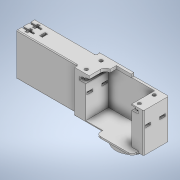
# Autodesk Inventor part: мотор_плеча_2.1-локтя_1
Saved by Autodesk Inventor 2022 (Build 260153000, 153)
## iProperties
Created: 2022-12-03
Part Number: мотор_плеча_2.1-локтя_1
Material: Типовые
Document SubType Name: Modeling
Designer: Папа
Density: 1 g/cm^3
Appearance: По умолчанию
Author: Папа
Autodesk Inventor part; units mm, degrees
ref_plane "YZ Plane" through (0, 0, 0) normal (1, 0, 0) x (0, 1, 0)
ref_plane "XZ Plane" through (0, 0, 0) normal (0, 1, 0) x (-1, 0, 0)
ref_plane "XY Plane" through (0, 0, 0) normal (0, 0, 1) x (1, 0, 0)
sketch "Эскиз1" plane through (0, 0, 0) normal (0, 1, 0) x (-1, 0, 0)
  line L0 (0, 0) -> (-59.05, 0)
  line L1 (-59.05, 0) -> (-59.05, -29.25)
  line L2 (-59.05, -29.25) -> (0, -29.25)
  line L3 (0, -29.25) -> (0, 0)
  line L4 (-74.05, 3) -> (15, 3)
  line L5 (15, 3) -> (15, -32.25)
  line L6 (15, -32.25) -> (-74.05, -32.25)
  line L7 (-74.05, -32.25) -> (-74.05, 3)
  line L8 (-74.05, 3) -> (15, -32.25) construction
  line L9 (15, 3) -> (-74.05, -32.25) construction
  line L10 (0, -29.25) -> (-59.05, 0) construction
  line L11 (0, 0) -> (-59.05, -29.25) construction
  line L12 (15, 0) -> (-74.05, 0)
  point P0 (-29.525, -14.625)
  point P1 (-29.525, -14.625)
  point P2 (-59.05, 0)
  point P3 (-59.05, 0)
  point P4 (0, 0)
  dimension "d0" = 29.25
  dimension "d1" = 59.05
  dimension "d2" = 15
  dimension "d3" = 3
  constraints: 26 end point, 4 midpoint, 4 parallel, 3 point on line, 2 horizontal, 2 perpendicular, 1 collinear
  measures "d0" distance of L2.end L0.start
  measures "d1" distance of L1.end L2.end
  measures "d2" distance between parallel lines of L3 L5
  measures "d3" distance between parallel lines of L6 L2
extrude "Выдавливание1" add sketch "Эскиз1" along normal blind 41 contours L12 L5 L6 L7 L1 L2 L3
sketch "Эскиз2" plane through (0, 0, 0) normal (0, -1, 0) x (1, 0, 0)
  line L0 (74.05, 0) -> (74.05, -32.25) projected
  line L1 (-15, -32.25) -> (-15, 0) projected
  line L2 (74.05, 0) -> (-15, 0)
  line L3 (-15, 0) -> (-15, -32.25)
  line L4 (-15, -32.25) -> (74.05, -32.25)
  line L5 (74.05, -32.25) -> (74.05, 0)
  point P0 (0, 0)
  constraints: 8 end point, 2 parallel, 1 horizontal, 1 perpendicular
extrude "Выдавливание2" add sketch "Эскиз2" along normal blind 2
sketch "Эскиз3" plane through (0, 41, 0) normal (0, 1, 0) x (1, 0, 0)
  circle A0 centre (-4.475, 5.225) radius 2.1
  circle A1 centre (-4.475, 24.225) radius 2.1
  circle A2 centre (63.525, 24.225) radius 2.1
  circle A3 centre (63.525, 5.225) radius 2.1
  line L0 (59.05, 29.25) -> (59.05, 0) construction
  line L1 (0, 0) -> (0, 29.25) construction
  line L2 (59.05, 29.25) -> (0, 29.25) construction
  line L3 (0, 29.25) -> (0, 0.2) construction
  line L4 (0, 0.2) -> (59.05, 0.2) construction
  line L5 (59.05, 0.2) -> (59.05, 29.25) construction
  line L6 (0, 0) -> (59.05, 0) construction
  line L7 (59.05, 0) -> (59.05, 0.2) construction
  line L8 (59.05, 0.2) -> (0, 0.2) construction
  line L9 (0, 0.2) -> (0, 0) construction
  line L10 (0, 0.2) -> (59.05, 29.25) construction
  line L11 (59.05, 0.2) -> (0, 29.25) construction
  line L12 (-4.475, 5.225) -> (63.525, 5.225) construction
  line L13 (63.525, 5.225) -> (63.525, 24.225) construction
  line L14 (63.525, 24.225) -> (-4.475, 24.225) construction
  line L15 (-4.475, 24.225) -> (-4.475, 5.225) construction
  line L16 (-4.475, 5.225) -> (63.525, 24.225) construction
  line L17 (-4.475, 24.225) -> (63.525, 5.225) construction
  point P0 (29.525, 14.725)
  dimension "d8" = 4.2
  dimension "d70" = 0.2
  dimension "d72" = 19
  dimension "d73" = 68
  constraints: 32 end point, 6 parallel, 4 centre point, 3 equal radius, 3 horizontal, 3 perpendicular, 2 coincident, 2 midpoint, 1 point on line
  measures "d8" diameter of A0
  measures "d70" distance between parallel lines of L4 L6
  measures "d72" distance of L13.end A3.centre
  measures "d73" distance of L13.end L14.end
extrude "Выдавливание3" cut sketch "Эскиз3" against normal blind 20
ref_plane "РабПлоскость1" through (0, 31, 0) normal (0, 1, 0) x (1, 0, 0)
sketch "Эскиз4" plane through (0, 31, 0) normal (0, 1, 0) x (1, 0, 0)
  circle A0 centre (63.525, 24.225) radius 2.1 projected
  line L0 (65.589, 27.8) -> (67.6531, 24.225)
  line L1 (67.6531, 24.225) -> (65.589, 20.65)
  line L2 (65.589, 20.65) -> (61.461, 20.65)
  line L3 (61.461, 20.65) -> (59.3969, 24.225)
  line L4 (59.3969, 24.225) -> (61.461, 27.8)
  line L5 (61.461, 27.8) -> (65.589, 27.8)
  circle A1 centre (-4.475, 24.225) radius 2.1 construction
  circle A2 centre (63.525, 5.225) radius 2.1 projected
  line L6 (-4.475, 24.225) -> (63.525, 24.225) construction
  line L7 (63.525, 24.225) -> (63.525, 5.225) construction
  line L8 (63.525, 5.225) -> (-4.475, 5.225) construction
  line L9 (-4.475, 5.225) -> (-4.475, 24.225) construction
  line L10 (-2.411, 27.8) -> (-0.3469, 24.225)
  line L11 (-0.3469, 24.225) -> (-2.411, 20.65)
  line L12 (-2.411, 20.65) -> (-6.539, 20.65)
  line L13 (-6.539, 20.65) -> (-8.6031, 24.225)
  line L14 (-8.6031, 24.225) -> (-6.539, 27.8)
  line L15 (-6.539, 27.8) -> (-2.411, 27.8)
  line L16 (65.589, 8.8) -> (67.6531, 5.225)
  line L17 (67.6531, 5.225) -> (65.589, 1.65)
  line L18 (65.589, 1.65) -> (61.461, 1.65)
  line L19 (61.461, 1.65) -> (59.3969, 5.225)
  line L20 (59.3969, 5.225) -> (61.461, 8.8)
  line L21 (61.461, 8.8) -> (65.589, 8.8)
  line L22 (-2.411, 8.8) -> (-0.3469, 5.225)
  line L23 (-0.3469, 5.225) -> (-2.411, 1.65)
  line L24 (-2.411, 1.65) -> (-6.539, 1.65)
  line L25 (-6.539, 1.65) -> (-8.6031, 5.225)
  line L26 (-8.6031, 5.225) -> (-6.539, 8.8)
  line L27 (-6.539, 8.8) -> (-2.411, 8.8)
  line L28 (65.589, 27.8) -> (74.05, 27.8)
  line L29 (74.05, 32.25) -> (74.05, 0) projected
  line L30 (65.589, 20.65) -> (74.05, 20.65)
  line L31 (29.525, 5.225) -> (29.525, 29.25) construction
  line L32 (0, 29.25) -> (59.05, 29.25) construction
  line L33 (0, 0) -> (0, 29.25) projected
  line L34 (0, 14.625) -> (59.05, 14.625) construction
  line L35 (59.05, 29.25) -> (59.05, 0) projected
  line L36 (59.05, 14.625) -> (0, 14.625) construction
  line L37 (-15, 27.8) -> (-15, 20.65)
  line L38 (-15, 0) -> (-15, 32.25) projected
  line L39 (65.589, 8.8) -> (74.05, 8.8)
  line L40 (65.589, 1.65) -> (74.05, 1.65)
  line L41 (74.05, 1.65) -> (74.05, 8.8)
  line L42 (-2.411, 27.8) -> (0, 27.8)
  line L43 (-2.411, 20.65) -> (0, 20.65)
  line L44 (0, 20.65) -> (0, 27.8)
  line L45 (-2.411, 8.8) -> (0, 8.8)
  line L46 (-2.411, 1.65) -> (0, 1.65)
  line L47 (0, 8.8) -> (0, 1.65)
  point P0 (-4.475, 24.225)
  point P1 (-4.475, 24.225)
  point P2 (63.525, 5.225)
  point P3 (63.525, 5.225)
  point P4 (-4.475, 5.225)
  point P5 (-4.475, 5.225)
  point P6 (-15, 1.45)
  point P7 (-15, 8.6)
  dimension "d14" = 7.15
  dimension "d17" = 68
  dimension "d20" = 19
  constraints: 86 end point, 8 point on line, 7 perpendicular, 6 symmetric about line, 4 collinear, 4 horizontal, 4 midpoint, 3 parallel, 1 coincident, 1 vertical, 55 other
  measures "d14" distance between parallel lines of L1 L4
  measures "d17" distance of point (63.525, 24.225) point (-4.475, 24.225)
  measures "d20" distance of point (63.525, 24.225) point (63.525, 5.225)
extrude "Выдавливание4" cut sketch "Эскиз4" against normal blind 3.25 contours A0 | L28 L29 L30 L1 L0 | L0 L1 L2 L3 L4 L5 | A2 | L42 L33 L43 L11 L10 | L10 L11 L12 L13 L14 L15 | L39 L29 L40 L17 L16 | L16 L17 L18 L19 L20 L21 | L45 L33 L46 L23 L22 | L22 L23 L24 L25 L26 L27
ref_plane "РабПлоскость2" through (0, 19.5, 0) normal (0, -1, 0) x (1, 0, 0)
ref_plane "РабПлоскость3" through (29.525, 41, -32.25) normal (-1, 0, 0) x (0, 0, 1)
ref_plane "РабПлоскость5" through (74.05, 41, 0) normal (0, -1, 0) x (-1, 0, 0)
sketch "Эскиз10" plane through (0, 41, 0) normal (0, 1, 0) x (1, 0, 0)
  line L0 (59.05, 0) -> (74.05, 0) projected
  line L1 (74.05, 32.25) -> (-15, 32.25) projected
  line L2 (74.05, 0) -> (-15, 0)
  line L3 (-15, 0) -> (-15, 32.25)
  line L4 (-15, 32.25) -> (74.05, 32.25)
  line L5 (74.05, 32.25) -> (74.05, 0)
  line L6 (0, 0) -> (0, 29.25) projected
  line L7 (59.05, 29.25) -> (59.05, 0) projected
  line L8 (0, 29.25) -> (59.05, 29.25)
  line L9 (59.05, 29.25) -> (59.05, 0)
  line L10 (59.05, 0) -> (0, 0)
  line L11 (0, 0) -> (0, 29.25)
  circle A0 centre (63.525, 24.225) radius 2.1 projected
  circle A1 centre (63.525, 24.225) radius 2.05
  circle A2 centre (63.525, 5.225) radius 2.05
  circle A3 centre (-4.475, 5.225) radius 2.1 projected
  circle A4 centre (-4.475, 5.225) radius 2.05
  circle A5 centre (-4.475, 24.225) radius 2.05
  circle A6 centre (-4.475, 24.225) radius 2.1 projected
  circle A7 centre (63.525, 5.225) radius 2.1 projected
  point P0 (74.05, 32.25)
  constraints: 16 end point, 6 coincident, 4 centre point, 4 parallel, 2 horizontal, 2 perpendicular
extrude "Выдавливание10" add sketch "Эскиз10" along normal blind 7 contours L7 L8 L6 L2 L3 L1 L5 L0 | A6 | A7
sketch "Эскиз11" plane through (74.05, 41, 0) normal (0, -1, 0) x (-1, 0, 0)
  line L0 (15, 29.25) -> (15, 0) projected
  line L1 (15, 0) -> (6.9, 0)
  line L2 (6.9, 0) -> (6.9, 29.05)
  line L3 (6.9, 29.05) -> (15, 29.05)
  line L4 (15, 29.05) -> (15, 0)
  point P0 (74.05, 0)
  point P1 (15, 29.05)
  dimension "d61" = 8.1
  constraints: 8 end point, 2 parallel, 1 horizontal, 1 perpendicular
  measures "d61" distance between parallel lines of L0 L2
extrude "Выдавливание11" cut sketch "Эскиз11" against normal blind 4
fillet "Сопряжение8" radius 1.95 1 edges at (67.15, 43, -29.05)
sketch "Эскиз13" plane through (74.05, 45, 0) normal (0, -1, 0) x (1, 0, 0)
  line L0 (-15, -29.25) -> (-15, 0) projected
  line L1 (-74.05, -29.25) -> (-15, -29.25) projected
  line L2 (-15, 0) -> (-15, -29.25)
  line L3 (-20, -13.625) -> (-10, -13.625)
  line L4 (-10, -13.625) -> (-10, -15.625)
  line L5 (-10, -15.625) -> (-20, -15.625)
  line L6 (-20, -15.625) -> (-20, -13.625)
  line L7 (-20, -13.625) -> (-10, -15.625) construction
  line L8 (-10, -13.625) -> (-20, -15.625) construction
  arc A0 (-11, -15.625) -> (-11, -13.625) centre (-11, -14.625) ccw
  line L9 (-10, -14.625) -> (-15, -14.625)
  line L10 (-15, -14.625) -> (-15, 0)
  line L11 (-15, 0) -> (-10, 0)
  line L12 (-10, 0) -> (-10, -14.625)
  point P0 (-74.05, 0)
  point P1 (-15, -13.625)
  dimension "d65" = 10
  dimension "d66" = 2
  constraints: 22 end point, 4 parallel, 3 midpoint, 3 point on circle, 3 tangent, 2 horizontal, 2 perpendicular, 2 point on line, 1 centre point, 1 vertical
  measures "d65" distance of L4.end L5.end
  measures "d66" distance of L3.end L4.end
extrude "Выдавливание12" cut sketch "Эскиз13" against normal blind 1.5
fillet "Сопряжение9" radius 1 1 edges at (64.05, 45.75, -15.625)
mirror "Зеркальное отражение2" about plane through (29.525, 41, -32.25) normal (-1, 0, 0) of "Выдавливание11", "Выдавливание12", "Сопряжение9"
sketch "Эскиз15" plane through (0, 48, 0) normal (0, 1, 0) x (1, 0, 0)
  arc A0 (42.1128, 0.625) -> (42.1128, 28.725) centre (44.775, 14.675) ccw
  line L0 (42.1128, 28.725) -> (10.5328, 28.725)
  line L1 (10.5328, 0.625) -> (42.1128, 0.625)
  arc A1 (10.5328, 20.7) -> (10.5328, 8.65) centre (10.5328, 14.675) ccw
  line L2 (10.5328, 28.725) -> (10.5328, 20.7)
  line L3 (10.5328, 8.65) -> (10.5328, 0.625)
  line L4 (-7.975, 29.225) -> (67.025, 29.225)
  line L5 (67.025, 29.225) -> (67.025, 0.125)
  line L6 (67.025, 0.125) -> (-7.975, 0.125)
  line L7 (-7.975, 0.125) -> (-7.975, 29.225)
  line L8 (-7.975, 29.225) -> (67.025, 0.125) construction
  line L9 (67.025, 29.225) -> (-7.975, 0.125) construction
  line L10 (59.075, 14.675) -> (67.025, 14.675)
  line L11 (10.5328, 20.7) -> (10.5328, 8.65) construction
  line L12 (67.025, 0.125) -> (-7.975, 0.125)
  line L13 (-7.975, 0.125) -> (-7.975, -2.875)
  line L14 (-7.975, -2.875) -> (67.025, -2.875)
  line L15 (67.025, -2.875) -> (67.025, 0.125)
  circle A2 centre (63.525, 24.225) radius 2.05
  circle A3 centre (63.525, 24.225) radius 2.1 projected
  circle A4 centre (-4.475, 24.225) radius 2.1 projected
  circle A5 centre (-4.475, 24.225) radius 2.1
  circle A6 centre (-4.475, 5.225) radius 2.1 projected
  circle A7 centre (-4.475, 5.225) radius 2.1
  circle A8 centre (63.525, 5.225) radius 2.05 projected
  circle A9 centre (63.525, 5.225) radius 2.05
  line L16 (4.5078, 14.675) -> (4.5078, 0)
  line L17 (59.05, 0) -> (0, 0) projected
  line L18 (29.525, 14.675) -> (29.525, 0)
  line L19 (74.05, 32.25) -> (-15, 32.25) projected
  line L20 (-15, 32.25) -> (29.525, 32.25)
  line L21 (29.525, 32.25) -> (29.525, 0)
  line L22 (29.525, 0) -> (-15, 0)
  line L23 (-15, 0) -> (-15, 32.25)
  point P0 (-52.75, -14.55)
  point P1 (29.525, 32.25)
  point P2 (-7.975, 0)
  point P3 (-7.975, 0.125)
  point P4 (4.5078, 0.125)
  point P5 (29.525, 28.725)
  dimension "d75" = 28.6
  dimension "d76" = 12.05
  dimension "d77" = 31.58
  dimension "d79" = 29.1
  dimension "d80" = 75
  dimension "d81" = 3
  dimension "d82" = 22.25
  dimension "d83" = 3.5
  dimension "d84" = 5
  dimension "d85" = 4.1
  dimension "d86" = 7.95
  dimension "d87" = 28.1
  constraints: 44 end point, 8 parallel, 6 centre point, 6 coincident, 6 point on circle, 5 horizontal, 5 perpendicular, 4 collinear, 4 midpoint, 1 point on line, 1 vertical
  measures "d75" diameter of A0
  measures "d76" diameter of A1
  measures "d77" distance of L1.start L1.end
  measures "d79" distance between parallel lines of L4 L6
  measures "d80" distance of L5.end L6.end
  measures "d81" distance of L14.end L5.end
  measures "d82" distance from line of L5 point (44.775, 14.675)
  measures "d83" distance from line of L5 A2.centre
  measures "d84" distance from line of L4 A2.centre
  measures "d85" diameter of A2
  measures "d86" distance of L10.start L10.end
  measures "d87" distance between parallel lines of L1 L0
extrude "Выдавливание13" add sketch "Эскиз15" along normal blind 4 contours L0 L2 A1 L16 L6 L7 L4 L21 | L16 L17 L22 L13 L6 | L4 L7 L13 L22 L23 L19 L21
sketch "Эскиз17" plane through (0, -2, 0) normal (0, -1, 0) x (1, 0, 0)
  circle A0 centre (63.525, -5.225) radius 2.05 projected
  circle A1 centre (63.525, -24.225) radius 2.1 projected
  line L0 (63.525, -5.225) -> (63.525, -24.225) construction
  line L1 (63.525, -14.725) -> (44.775, -14.725) construction
  circle A2 centre (44.775, -14.725) radius 18.9
  circle A3 centre (44.775, -14.725) radius 20.9
  point P0 (0, 0)
  dimension "d92" = 18.75
  dimension "d93" = 37.8
  dimension "d94" = 2
  constraints: 4 end point, 2 centre point, 2 coincident, 1 horizontal, 1 midpoint, 1 vertical
  measures "d92" distance of L1.start L1.end
  measures "d93" diameter of A2
  measures "d94" radial gap between concentric circles of A3 A2
extrude "Выдавливание15" add sketch "Эскиз17" along normal blind 6 contours A3 A0 | A0 A3 A1 | A1 A3 picked at (62.8379, -5.5731) picked at (62.8227, -23.8692)
sketch "Эскиз18" plane through (44.775, -8, -14.725) normal (0, -1, 0) x (1, 0, 0)
  circle A0 centre (0, 0) radius 18.9 projected
  circle A1 centre (-18.9, 0) radius 0.25
  line L0 (0, 0) -> (-17.8021, 0) construction
  point P0 (-44.775, 14.725)
  dimension "d99" = 0.5
  constraints: 2 end point, 1 centre point, 1 horizontal, 1 horizontal alignment, 1 other
  measures "d99" diameter of A1
extrude "Выдавливание16" add sketch "Эскиз18" against normal up to surface (6 mm away) contours A1 A0 | A0 A1 picked at (-18.8165, 0) picked at (-18.9826, -0.0101)
fillet "Сопряжение12" radius 0.7 2 edges at (25.8767, -5, -14.475) (25.8767, -5, -14.975)
pattern_circular "Круговой массив1" count 12 over 360 about axis through (44.775, -2, -14.725) along (0, -1, 0) of "Выдавливание16", "Сопряжение12"
fillet "Сопряжение14" radius 1.5 2 edges at (74.05, 23, 0) (74.05, 23, -32.25)
sketch "Эскиз27" plane through (-15, -2, -32.25) normal (-1, 0, 0) x (0, 0, 1)
  line L0 (32.25, 0) -> (32.25, 54) projected
  line L1 (0, 54) -> (32.25, 54) projected
  line L2 (0, 0) -> (0, 54) projected
  line L3 (32.25, 0) -> (0, 0) projected
  line L4 (0, 54) -> (32.25, 54) projected
  line L5 (16.125, 54) -> (16.125, 27) construction
  line L6 (28.125, 54) -> (4.125, 54)
  line L7 (4.125, 54) -> (4.125, 0)
  line L8 (4.125, 0) -> (28.125, 0)
  line L9 (28.125, 0) -> (28.125, 54)
  line L10 (28.125, 54) -> (4.125, 0) construction
  line L11 (4.125, 54) -> (28.125, 0) construction
  point P0 (32.25, 2)
  point P1 (4.125, 54)
  dimension "d148" = 27
  dimension "d149" = 24
  constraints: 14 end point, 3 midpoint, 2 parallel, 1 horizontal, 1 perpendicular, 1 point on line, 1 vertical
  measures "d148" distance of L5.start L5.end
  measures "d149" distance between parallel lines of L7 L9
extrude "Выдавливание24" add sketch "Эскиз27" along normal blind 50 contours L3 L7 L1 L9
sketch "Эскиз28" plane through (-65, -2, -32.25) normal (-1, 0, 0) x (0, 0, 1)
  line L0 (28.125, 54) -> (4.125, 54) projected
  line L1 (4.125, 54) -> (4.125, 0) projected
  line L2 (4.125, 0) -> (28.125, 0) projected
  line L3 (28.125, 0) -> (28.125, 54) projected
  line L4 (4.125, 0) -> (4.125, 54) projected
  line L5 (28.125, 0) -> (4.125, 54) construction
  line L6 (26.175, 47.05) -> (6.075, 47.05)
  line L7 (6.075, 47.05) -> (6.075, 6.95)
  line L8 (6.075, 6.95) -> (26.175, 6.95)
  line L9 (26.175, 6.95) -> (26.175, 47.05)
  line L10 (26.175, 47.05) -> (6.075, 6.95) construction
  line L11 (6.075, 47.05) -> (26.175, 6.95) construction
  point P0 (32.25, 2)
  point P1 (16.125, 27)
  dimension "d152" = 40.1
  dimension "d153" = 20.1
  constraints: 14 end point, 3 midpoint, 2 parallel, 1 horizontal, 1 perpendicular
  measures "d152" distance between parallel lines of L6 L8
  measures "d153" distance between parallel lines of L9 L7
extrude "Выдавливание25" add sketch "Эскиз28" along normal blind 27.5
sketch "Эскиз29" plane through (-92.5, -2, -32.25) normal (-1, 0, 0) x (0, 0, 1)
  line L0 (4.125, 54) -> (4.125, 0) construction
  line L1 (4.125, 0) -> (28.125, 0) construction
  line L2 (28.125, 0) -> (28.125, 54) construction
  line L3 (28.125, 54) -> (4.125, 54) construction
  line L4 (26.175, 47.05) -> (26.175, 6.95) construction
  line L5 (26.175, 6.95) -> (6.075, 6.95) construction
  line L6 (6.075, 6.95) -> (6.075, 47.05) construction
  line L7 (6.075, 47.05) -> (26.175, 47.05) construction
  line L8 (32.25, 0) -> (28.125, 0) construction
  line L9 (28.125, 0) -> (4.125, 54) construction
  line L10 (20.875, 52.2) -> (11.375, 52.2) construction
  line L11 (11.375, 52.2) -> (11.375, 1.8) construction
  line L12 (11.375, 1.8) -> (20.875, 1.8) construction
  line L13 (20.875, 1.8) -> (20.875, 52.2) construction
  line L14 (20.875, 52.2) -> (11.375, 1.8) construction
  line L15 (11.375, 52.2) -> (20.875, 1.8) construction
  circle A0 centre (11.375, 52.2) radius 2.05
  circle A1 centre (20.875, 52.2) radius 2.05
  circle A2 centre (20.875, 1.8) radius 2.05
  circle A3 centre (11.375, 1.8) radius 2.05
  point P0 (32.25, 2)
  point P1 (16.125, 27)
  dimension "d156" = 9.5
  dimension "d157" = 50.4
  dimension "d158" = 4.1
  constraints: 14 end point, 4 centre point, 4 coincident, 3 equal radius, 3 midpoint, 2 parallel, 1 horizontal, 1 perpendicular
  measures "d156" distance of L11.end L12.end
  measures "d157" distance of L10.end L11.end
  measures "d158" diameter of A0
extrude "Выдавливание26" cut sketch "Эскиз29" against normal blind 15
ref_plane "РабПлоскость8" through (-82.5, -2, -32.25) normal (-1, 0, 0) x (0, 0, 1)
sketch "Эскиз30" plane through (-82.5, -2, -32.25) normal (-1, 0, 0) x (0, 0, 1)
  arc A0 (21.8561, 0) -> (19.8939, 0) centre (20.875, 1.8) ccw construction
  arc A1 (12.3561, 0) -> (10.3939, 0) centre (11.375, 1.8) ccw construction
  arc A2 (10.3939, 54) -> (12.3561, 54) centre (11.375, 52.2) ccw construction
  line L0 (20.875, 1.8) -> (11.375, 1.8) construction
  line L1 (32.25, 2) -> (3, 2) construction
  line L2 (11.375, 1.8) -> (11.375, 52.2) construction
  line L3 (11.375, -2.2415) -> (7.875, -0.2207)
  line L4 (7.875, -0.2207) -> (7.875, 3.8207)
  line L5 (7.875, 3.8207) -> (11.375, 5.8415)
  line L6 (11.375, 5.8415) -> (14.875, 3.8207)
  line L7 (14.875, 3.8207) -> (14.875, -0.2207)
  line L8 (14.875, -0.2207) -> (11.375, -2.2415)
  line L9 (20.875, -2.2415) -> (17.375, -0.2207)
  line L10 (17.375, -0.2207) -> (17.375, 3.8207)
  line L11 (17.375, 3.8207) -> (20.875, 5.8415)
  line L12 (20.875, 5.8415) -> (24.375, 3.8207)
  line L13 (24.375, 3.8207) -> (24.375, -0.2207)
  line L14 (24.375, -0.2207) -> (20.875, -2.2415)
  line L15 (11.375, 48.1585) -> (7.875, 50.1793)
  line L16 (7.875, 50.1793) -> (7.875, 54.2207)
  line L17 (7.875, 54.2207) -> (11.375, 56.2415)
  line L18 (11.375, 56.2415) -> (14.875, 54.2207)
  line L19 (14.875, 54.2207) -> (14.875, 50.1793)
  line L20 (14.875, 50.1793) -> (11.375, 48.1585)
  line L21 (20.875, 48.1585) -> (17.375, 50.1793)
  line L22 (17.375, 50.1793) -> (17.375, 54.2207)
  line L23 (17.375, 54.2207) -> (20.875, 56.2415)
  line L24 (20.875, 56.2415) -> (24.375, 54.2207)
  line L25 (24.375, 54.2207) -> (24.375, 50.1793)
  line L26 (24.375, 50.1793) -> (20.875, 48.1585)
  point P0 (20.875, 52.2)
  dimension "d162" = 7
  dimension "d165" = 9.5
  dimension "d168" = 50.4
  constraints: 52 end point, 2 vertical, 1 coincident, 1 horizontal, 1 parallel, 1 perpendicular, 52 other
  measures "d162" distance between parallel lines of L7 L4
  measures "d165" distance of point (11.375, 1.8) point (20.875, 1.8)
  measures "d168" distance of point (11.375, 1.8) point (11.375, 52.2)
extrude "Выдавливание27" cut sketch "Эскиз30" along normal blind 3.3
sketch "Эскиз31" plane through (0, 52, 0) normal (0, 1, 0) x (1, 0, 0)
  line L0 (-85.8, 17.375) -> (-85.8, 19.8939) construction
  line L1 (-85.8, 19.8939) -> (-92.5, 19.8939) construction
  line L2 (-92.5, 12.3561) -> (-92.5, 19.8939) construction
  line L3 (-92.5, 12.3561) -> (-85.8, 12.3561) construction
  line L4 (-85.8, 12.3561) -> (-85.8, 14.875) construction
  line L5 (-85.8, 14.875) -> (-82.5, 14.875) construction
  line L6 (-82.5, 14.875) -> (-82.5, 12.3561) construction
  line L7 (-82.5, 12.3561) -> (-77.5, 12.3561) construction
  line L8 (-77.5, 12.3561) -> (-77.5, 10.3939) construction
  line L9 (-77.5, 10.3939) -> (-82.5, 10.3939) construction
  line L10 (-82.5, 10.3939) -> (-82.5, 7.875) construction
  line L11 (-82.5, 7.875) -> (-85.8, 7.875) construction
  line L12 (-85.8, 7.875) -> (-85.8, 10.3939) construction
  line L13 (-85.8, 10.3939) -> (-92.5, 10.3939) construction
  line L14 (-92.5, 4.125) -> (-92.5, 10.3939) construction
  line L15 (-15, 4.125) -> (-92.5, 4.125) construction
  line L16 (-15, 4.125) -> (-15, 0) construction
  line L17 (-15, 0) -> (4.5078, 0) construction
  line L18 (4.5078, 0) -> (4.5078, 14.675) construction
  arc A0 (10.5328, 20.7) -> (4.5078, 14.675) centre (10.5328, 14.675) ccw construction
  line L19 (10.5328, 20.7) -> (10.5328, 28.725) construction
  line L20 (10.5328, 28.725) -> (29.525, 28.725) construction
  line L21 (29.525, 28.725) -> (29.525, 32.25) construction
  line L22 (29.525, 32.25) -> (-15, 32.25) construction
  line L23 (-15, 32.25) -> (-15, 28.125) construction
  line L24 (-15, 28.125) -> (-92.5, 28.125) construction
  line L25 (-92.5, 21.8561) -> (-92.5, 28.125) construction
  line L26 (-92.5, 21.8561) -> (-85.8, 21.8561) construction
  line L27 (-85.8, 21.8561) -> (-85.8, 24.375) construction
  line L28 (-85.8, 24.375) -> (-82.5, 24.375) construction
  line L29 (-82.5, 24.375) -> (-82.5, 21.8561) construction
  line L30 (-82.5, 21.8561) -> (-77.5, 21.8561) construction
  line L31 (-77.5, 21.8561) -> (-77.5, 19.8939) construction
  line L32 (-77.5, 19.8939) -> (-82.5, 19.8939) construction
  line L33 (-82.5, 19.8939) -> (-82.5, 17.375) construction
  line L34 (-82.5, 17.375) -> (-85.8, 17.375) construction
  circle A1 centre (-4.475, 5.225) radius 2.1 construction
  circle A2 centre (-4.475, 24.225) radius 2.1 construction
  line L35 (-15, 28.125) -> (-15, 32.25) construction
  line L36 (-92.5, 10.3939) -> (-92.5, 4.125) construction
  line L37 (-15, 28.125) -> (-92.5, 28.125) construction
  line L38 (-92.5, 28.125) -> (-92.5, 4.125) construction
  line L39 (-92.5, 4.125) -> (-15, 4.125) construction
  line L40 (-15, 4.125) -> (-15, 28.125) construction
  line L41 (-15, 16.125) -> (-70, 16.125) construction
  line L42 (-70, 16.125) -> (-70, 28.125) construction
  line L43 (-15, 28.125) -> (-92.5, 28.125) construction
  line L44 (-71.75, 19.625) -> (-68.25, 19.625)
  line L45 (-68.25, 19.625) -> (-68.25, 12.625)
  line L46 (-68.25, 12.625) -> (-71.75, 12.625)
  line L47 (-71.75, 12.625) -> (-71.75, 19.625)
  line L48 (-71.75, 19.625) -> (-68.25, 12.625) construction
  line L49 (-68.25, 19.625) -> (-71.75, 12.625) construction
  dimension "d173" = 55
  dimension "d174" = 3.5
  dimension "d175" = 7
  constraints: 24 end point, 4 parallel, 3 horizontal, 3 midpoint, 3 perpendicular, 1 point on line
  measures "d173" distance of L41.start L41.end
  measures "d174" distance of L45.end L46.end
  measures "d175" distance of L46.end L44.start
extrude "Выдавливание28" cut sketch "Эскиз31" against normal blind 10
sketch "Эскиз32" plane through (-92.5, -2, -32.25) normal (-1, 0, 0) x (0, 0, 1)
  line L0 (19.625, 54) -> (12.625, 54) projected
  line L1 (6.075, 47.05) -> (26.175, 47.05) projected
  line L2 (12.625, 54) -> (12.625, 47.05)
  line L3 (12.625, 54) -> (12.625, 47.05) projected
  line L4 (19.625, 54) -> (19.625, 47.05)
  line L5 (19.625, 54) -> (19.625, 47.05) projected
  line L6 (12.625, 47.05) -> (19.625, 47.05)
  line L7 (19.625, 47.05) -> (19.625, 48.55)
  line L8 (19.625, 48.55) -> (12.625, 48.55)
  line L9 (12.625, 48.55) -> (12.625, 47.05)
  point P0 (32.25, 2)
  point P1 (12.625, 44)
  point P2 (19.625, 44)
  dimension "d178" = 1.5
  constraints: 14 end point, 3 point on line, 2 parallel, 1 horizontal, 1 perpendicular
  measures "d178" distance between parallel lines of L1 L8
extrude "Выдавливание29" cut sketch "Эскиз32" against normal up to surface (24.25 mm away) contours L4 L1 L2 L8
sketch "Эскиз33" plane through (0, -2, 0) normal (0, -1, 0) x (1, 0, 0)
  arc A0 (29.9431, 0) -> (33.3871, -32.25) centre (44.775, -14.725) ccw construction
  circle A1 centre (44.775, -14.725) radius 20.9 construction
  line L0 (23.875, -35.625) -> (65.675, -35.625) construction
  line L1 (65.675, -35.625) -> (65.675, 6.175) construction
  line L2 (65.675, 6.175) -> (23.875, 6.175) construction
  line L3 (23.875, 6.175) -> (23.875, -35.625) construction
  line L4 (23.875, -35.625) -> (65.675, 6.175) construction
  line L5 (65.675, -35.625) -> (23.875, 6.175) construction
  line L6 (21.875, -37.625) -> (67.675, -37.625)
  line L7 (67.675, -37.625) -> (67.675, 8.175)
  line L8 (67.675, 8.175) -> (21.875, 8.175)
  line L9 (21.875, 8.175) -> (21.875, -37.625)
  line L10 (21.875, -37.625) -> (67.675, 8.175) construction
  line L11 (67.675, -37.625) -> (21.875, 8.175) construction
  line L12 (59.05, 0) -> (0, 0) projected
  line L13 (74.05, -1.5) -> (74.05, -30.75) projected
  line L14 (14.1054, 0) -> (86.1611, 0) construction
  line L15 (74.05, -27.8) -> (74.05, -20.65) projected
  line L16 (74.05, -26.45) -> (74.05, 10.0078) construction
  circle A2 centre (44.775, -14.725) radius 32.7697 construction
  line L17 (29.9431, 0) -> (-15, 0) projected
  line L18 (21.875, 0) -> (67.675, 0)
  line L19 (59.05, 0) -> (72.55, 0) projected
  line L20 (56.1629, -32.25) -> (72.55, -32.25) projected
  line L21 (67.675, -32.25) -> (21.875, -32.25)
  line L22 (-15, -32.25) -> (33.3871, -32.25) projected
  point P0 (21.875, 0)
  dimension "d182" = 2
  constraints: 32 end point, 11 point on line, 4 midpoint, 4 parallel, 4 perpendicular, 2 centre point, 2 coincident, 2 horizontal, 1 collinear, 1 point on circle, 1 tangent
  measures "d182" distance between parallel lines of L8 L2
extrude "Выдавливание30" add sketch "Эскиз33" against normal up to surface (2 mm away) contours L9 L21 L20 L7 L6 | L9 L8 L7 L18 L12
fillet "Сопряжение18" radius 5 4 edges at (67.675, -1, -37.625) (21.875, -1, -37.625) (67.675, -1, 8.175) (21.875, -1, 8.175)
fillet "Сопряжение19" radius 1 14 edges at (-53.75, -2, -28.125) (-53.75, -2, -4.125) (-53.75, 52, -28.125) (-53.75, 52, -4.125) (-15, 25, -28.125) (-15, -2, -30.1875) (-15, 25, -4.125) (-15, -2, -2.0625) (-15, 25, -32.25) (3.4375, -2, -32.25) (-15, 25, 0) (-15, 52, -2.0625) (-15, 52, -30.1875) (3.4375, -2, 0)
sketch "Эскиз19" plane through (-15, -2, -32.25) normal (-1, 0, 0) x (0, 0, 1)
  line L0 (32.25, 0) -> (32.25, 54) projected
  line L1 (0, 54) -> (32.25, 54) projected
  line L2 (0, 0) -> (0, 54) projected
  line L3 (32.25, 0) -> (0, 0) projected
  line L4 (32.25, 0) -> (0, 0) projected
  line L5 (2.125, 0) -> (30.125, 0)
  line L6 (30.125, 0) -> (30.125, 47.7)
  line L7 (30.125, 47.7) -> (2.125, 47.7)
  line L8 (2.125, 47.7) -> (2.125, 0)
  line L9 (2.125, 23.85) -> (0, 23.85) construction
  line L10 (0, 0) -> (0, 54) projected
  line L11 (30.125, 23.85) -> (32.25, 23.85) construction
  point P0 (32.25, 2)
  dimension "d108" = 47.7
  dimension "d109" = 28
  constraints: 12 end point, 4 point on line, 2 collinear, 2 horizontal, 2 midpoint, 2 parallel, 1 perpendicular
  measures "d108" distance between parallel lines of L3 L7
  measures "d109" distance between parallel lines of L6 L8
sketch "Эскиз20" plane through (-21, -2, -32.25) normal (-1, 0, 0) x (0, 0, 1)
  line L0 (2.125, 47.7) -> (2.125, 0) projected
  line L1 (2.125, 0) -> (30.125, 0) projected
  line L2 (30.125, 0) -> (30.125, 47.7) projected
  line L3 (30.125, 47.7) -> (2.125, 47.7) projected
  line L4 (30.125, 0) -> (2.125, 47.7) construction
  line L5 (26.125, 43.7) -> (6.125, 43.7)
  line L6 (6.125, 43.7) -> (6.125, 4)
  line L7 (6.125, 4) -> (26.125, 4)
  line L8 (26.125, 4) -> (26.125, 43.7)
  line L9 (26.125, 43.7) -> (6.125, 4) construction
  line L10 (6.125, 43.7) -> (26.125, 4) construction
  point P0 (32.25, 2)
  point P1 (16.125, 23.85)
  dimension "d113" = 4
  dimension "d114" = 4
  constraints: 14 end point, 3 midpoint, 2 parallel, 1 horizontal, 1 perpendicular
  measures "d113" distance between parallel lines of L1 L7
  measures "d114" distance between parallel lines of L0 L6
sketch "Эскиз21" plane through (-21, -2, -32.25) normal (-1, 0, 0) x (0, 0, 1)
  line L0 (26.125, 43.7) -> (6.125, 43.7) construction
  line L1 (6.125, 43.7) -> (6.125, 4) construction
  line L2 (6.125, 4) -> (26.125, 4) construction
  line L3 (26.125, 4) -> (26.125, 43.7) construction
  line L4 (6.125, 4) -> (26.125, 4) construction
  line L5 (26.125, 4) -> (26.125, 43.7) construction
  line L6 (6.125, 4) -> (26.125, 43.7) construction
  line L7 (6.125, 43.7) -> (6.125, 4) construction
  line L8 (26.125, 4) -> (6.125, 43.7) construction
  line L9 (16.125, 4) -> (16.125, 23.85) construction
  circle A0 centre (16.125, 13.8) radius 3.075
  point P0 (32.25, 2)
  dimension "d117" = 9.8
  dimension "d118" = 6.15
  constraints: 6 end point, 2 midpoint, 1 centre point, 1 perpendicular, 1 point on line
  measures "d117" distance from line of L2 A0.centre
  measures "d118" diameter of A0
sketch "Эскиз22" plane through (-21, -2, -32.25) normal (-1, 0, 0) x (0, 0, 1)
  circle A0 centre (16.125, 13.8) radius 3.075 projected
  circle A1 centre (16.125, 13.8) radius 6.5
  point P0 (32.25, 2)
  dimension "d121" = 13
  constraints: 1 centre point, 1 coincident
  measures "d121" diameter of A1
sketch "Эскиз23" plane through (0, -2, 0) normal (0, -1, 0) x (1, 0, 0)
  line L0 (-21, -26.125) -> (-21, -6.125) projected
  line L1 (-21, -16.125) -> (-28.5, -16.125) construction
  line L2 (-28.5, -13.725) -> (-33, -13.725)
  line L3 (-33, -13.725) -> (-33, -18.525)
  line L4 (-33, -18.525) -> (-28.5, -18.525)
  line L5 (-28.5, -18.525) -> (-28.5, -13.725)
  line L6 (-21, -16.125) -> (-28.5, -18.525) construction
  line L7 (-28.5, -13.725) -> (-21, -16.125) construction
  point P0 (0, 0)
  dimension "d124" = 7.5
  dimension "d125" = 4.8
  dimension "d130" = 4.5
  constraints: 14 end point, 2 horizontal, 2 midpoint, 2 parallel, 1 equal length, 1 perpendicular
  measures "d124" distance of L1.start L1.end
  measures "d125" distance between parallel lines of L2 L4
  measures "d130" distance between parallel lines of L3 L5
sketch "Эскиз25" plane through (-56.2, -2, -32.25) normal (-1, 0, 0) x (0, 0, 1)
  line L0 (2.125, 0) -> (30.125, 0) construction
  line L1 (30.125, 0) -> (30.125, 47.7) construction
  line L2 (30.125, 47.7) -> (2.125, 47.7) construction
  line L3 (2.125, 47.7) -> (2.125, 0) construction
  line L4 (26.125, 43.7) -> (26.125, 4) construction
  line L5 (26.125, 4) -> (6.125, 4) construction
  line L6 (6.125, 4) -> (6.125, 43.7) construction
  line L7 (6.125, 43.7) -> (26.125, 43.7) construction
  line L8 (30.125, 47.7) -> (31.625, 49.2) construction
  line L9 (30.125, 47.7) -> (26.125, 43.7) construction
  line L10 (26.125, 4) -> (26.125, 43.7) construction
  line L11 (26.125, 4) -> (6.125, 43.7) construction
  line L12 (26.125, 43.7) -> (6.125, 4) construction
  line L13 (16.125, 23.85) -> (26.125, 23.85) construction
  line L14 (16.125, 23.85) -> (16.125, 43.7) construction
  line L15 (6.125, 43.7) -> (26.125, 43.7) construction
  circle A0 centre (27.7819, 45.3569) radius 2.3431 construction
  circle A1 centre (27.7819, 45.3569) radius 1.05
  circle A2 centre (4.4681, 45.3569) radius 1.05
  circle A3 centre (27.7819, 2.3431) radius 1.05
  circle A4 centre (4.4681, 2.3431) radius 1.05
  point P0 (32.25, 2)
  dimension "d131" = 2.1
  constraints: 10 end point, 4 centre point, 3 midpoint, 3 symmetric about line, 1 coincident, 1 collinear, 1 horizontal, 1 point on line, 6 other
  measures "d131" diameter of A1
sketch "Эскиз26" plane through (-46.2, -2, -32.25) normal (-1, 0, 0) x (0, 0, 1)
  circle A0 centre (21.0926, -11.2426) radius 1.05
  line L0 (2.125, 47.7) -> (30.125, 47.7) projected
  circle A1 centre (4.4681, 45.3569) radius 1.05 projected
  line L1 (6.1624, 47.0511) -> (6.7825, 44.7367)
  line L2 (6.7825, 44.7367) -> (5.0883, 43.0425)
  line L3 (5.0883, 43.0425) -> (2.7739, 43.6626)
  line L4 (2.7739, 43.6626) -> (2.1538, 45.977)
  line L5 (2.1538, 45.977) -> (3.848, 47.6712)
  line L6 (3.848, 47.6712) -> (6.1624, 47.0511)
  line L7 (26.125, 43.7) -> (6.125, 43.7) projected
  line L8 (6.7825, 44.7367) -> (9.7458, 47.7)
  line L9 (9.7458, 47.7) -> (6.8113, 50.6345)
  line L10 (6.8113, 50.6345) -> (3.848, 47.6712)
  circle A2 centre (4.4681, 2.3431) radius 1.05 projected
  circle A3 centre (4.4681, 45.3569) radius 1.05 projected
  circle A4 centre (27.7819, 45.3569) radius 1.05 projected
  circle A5 centre (27.7819, 2.3431) radius 1.05 projected
  line L11 (2.125, 0) -> (30.125, 0) projected
  line L12 (30.125, 0) -> (30.125, 47.7) projected
  line L13 (30.125, 47.7) -> (2.125, 47.7) projected
  line L14 (2.125, 47.7) -> (2.125, 0) projected
  line L15 (26.125, 43.7) -> (26.125, 4) projected
  line L16 (26.125, 4) -> (6.125, 4) projected
  line L17 (6.125, 4) -> (6.125, 43.7) projected
  line L18 (6.125, 43.7) -> (26.125, 43.7) projected
  line L19 (30.125, 47.7) -> (30.125, 0) projected
  line L20 (0.625, 0) -> (2.125, 0) projected
  line L21 (30.125, 47.7) -> (2.125, 0) construction
  line L22 (16.125, 23.85) -> (23.6976, 23.85) construction
  line L23 (16.125, 23.85) -> (16.125, 29.0933) construction
  circle A6 centre (27.7819, 45.3569) radius 1.05
  line L24 (26.0876, 47.0511) -> (25.4675, 44.7367)
  line L25 (25.4675, 44.7367) -> (27.1617, 43.0425)
  line L26 (27.1617, 43.0425) -> (29.4761, 43.6626)
  line L27 (29.4761, 43.6626) -> (30.0962, 45.977)
  line L28 (30.0962, 45.977) -> (28.402, 47.6712)
  line L29 (28.402, 47.6712) -> (26.0876, 47.0511)
  line L30 (25.4675, 44.7367) -> (22.5042, 47.7)
  line L31 (22.5042, 47.7) -> (25.4387, 50.6345)
  line L32 (25.4387, 50.6345) -> (28.402, 47.6712)
  circle A7 centre (27.7819, 45.3569) radius 1.05
  line L33 (2.125, 0) -> (30.125, 0)
  circle A8 centre (4.4681, 2.3431) radius 1.05
  line L34 (6.1624, 0.6489) -> (6.7825, 2.9633)
  line L35 (6.7825, 2.9633) -> (5.0883, 4.6575)
  line L36 (5.0883, 4.6575) -> (2.7739, 4.0374)
  line L37 (2.7739, 4.0374) -> (2.1538, 1.723)
  line L38 (2.1538, 1.723) -> (3.848, 0.0288)
  line L39 (3.848, 0.0288) -> (6.1624, 0.6489)
  line L40 (26.125, 4) -> (6.125, 4)
  line L41 (6.7825, 2.9633) -> (9.7458, 0)
  line L42 (9.7458, 0) -> (6.8113, -2.9345)
  line L43 (6.8113, -2.9345) -> (3.848, 0.0288)
  circle A9 centre (4.4681, 2.3431) radius 1.05
  circle A10 centre (27.7819, 2.3431) radius 1.05
  line L44 (30.125, 0) -> (2.125, 0)
  line L45 (6.125, 4) -> (26.125, 4)
  circle A11 centre (27.7819, 2.3431) radius 1.05
  circle A12 centre (27.7819, 2.3431) radius 1.05
  line L46 (25.4675, 2.9633) -> (27.1617, 4.6575)
  line L47 (25.4675, 2.9633) -> (22.5042, 0)
  line L48 (27.1617, 4.6575) -> (29.4761, 4.0374)
  line L49 (29.4761, 4.0374) -> (30.0962, 1.723)
  line L50 (30.0962, 1.723) -> (28.402, 0.0288)
  line L51 (26.0876, 0.6489) -> (25.4675, 2.9633)
  line L52 (22.5042, 0) -> (25.4387, -2.9345)
  line L53 (25.4387, -2.9345) -> (28.402, 0.0288)
  line L54 (28.402, 0.0288) -> (26.0876, 0.6489)
  point P0 (30.125, 47.7)
  point P1 (30.125, 47.7)
  point P2 (30.125, 0)
  point P3 (30.125, 0)
  dimension "d143" = 4.15
  dimension "d144" = 45
  constraints: 46 end point, 13 centre point, 11 coincident, 11 parallel, 11 tangent, 6 horizontal, 5 perpendicular, 1 vertical
  measures "d143" distance between parallel lines of L2 L5
  measures "d144" angle of L2 L7
